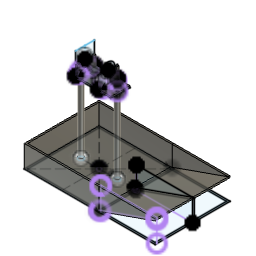
MiniFountain (Autodesk Fusion 360 design; units mm, degrees)
Autodesk Fusion 360 part; units mm, degrees
sketch "Base" plane through (0, 0, 0) normal (0, 0, 1) x (1, 0, 0)
  line L0 (70, 70) -> (-70, 70)
  line L1 (-70, 70) -> (-70, -70)
  line L2 (-70, -70) -> (70, -70)
  line L3 (70, -70) -> (70, 70)
  line L4 (70, 70) -> (-70, -70) construction
  line L5 (-70, 70) -> (70, -70) construction
  line L6 (-73.35, -73.35) -> (73.35, -73.35)
  line L7 (73.35, -73.35) -> (73.35, 73.35)
  line L8 (73.35, 73.35) -> (-73.35, 73.35)
  line L9 (-73.35, 73.35) -> (-73.35, -73.35)
  line L10 (70, 70) -> (180, 70)
  line L11 (70, -70) -> (180, -70)
  line L12 (180, -70) -> (180, 70)
  line L13 (70, 73.35) -> (183.35, 73.35)
  line L14 (183.35, -73.35) -> (183.35, 73.35)
  line L15 (70, -73.35) -> (183.35, -73.35)
  line L16 (0, 0) -> (-30.5813, 0)
  line L17 (0, 70) -> (0, -70) construction
  line L18 (0, 0) -> (30.5813, 0)
  circle A0 centre (-35.5812, 0.0143) radius 5
  circle A1 centre (35.5812, 0.0143) radius 5
  dimension "d5" = 140
  dimension "d6" = 140
  dimension "d8" = 3.35
  dimension "d9" = 110
  dimension "d10" = 110
  dimension "d16" = 30.5813
  dimension "d17" = 10
  constraint horizontal L0
  constraint perpendicular L0 L1
  constraint parallel L0 L2
  constraint parallel L1 L3
  constraint coincident L4 L16.start
  constraint coincident L5 L16.start
  constraint coincident L16.start L18.start
  constraint perpendicular L7 L10
  constraint perpendicular L7 L11
  constraint parallel L8 L16
  constraint midpoint L0 L17.start
  constraint midpoint L2 L17.end
  constraint symmetric L16.start L17 L18.start
  constraint symmetric L16.end L17 L18.end
  constraint coincident L16.end A0
  constraint symmetric L17 A0 A1
  measures "d5" distance of L1.end L2.end
  measures "d6" distance of L0.end L1.end
  measures "d9" distance of L0.start L10.end
  measures "d10" distance of L2.end L11.end
  measures "d16" distance of L16.start L16.end
  measures "d17" diameter of A0
extrude "Extrude1" add sketch "Base" along normal blind 43.35 contours L0 L1 L2 L6 L7 L8 L9 L10 L11 L13 L15 makes body 1
extrude "Extrude2" add sketch "Base" along normal blind 3.35 contours L0 L1 L2 L3 bodies 1
extrude "Extrude3" add sketch "Base" along normal blind 150 contours A0 | A1 bodies 1
sketch "Centered ramp wall" plane through (0, 0, 0) normal (0, 1, 0) x (1, 0, 0)
  line L0 (70, 0) -> (183.35, 0)
  line L1 (183.35, 0) -> (183.35, -43.35)
  line L2 (186.7, 0) -> (186.7, -43.35)
  line L3 (186.7, 0) -> (183.35, 0)
  line L4 (186.7, -43.35) -> (183.35, -43.35)
  line L5 (73.35, 0) -> (73.35, -43.35)
  line L6 (73.35, 0) -> (73.35, -43.35)
  line L7 (73.35, -43.35) -> (183.35, -43.35)
  line L8 (70, 0) -> (70, -3.35)
  line L9 (70, -3.35) -> (70, 0)
  line L10 (70, -3.35) -> (183.35, -43.35)
  line L11 (70, 0) -> (183.35, -40)
  dimension "d24" = 43.35
  constraint coincident L0.end L1.start
  constraint perpendicular L0 L1
  constraint perpendicular L1 L3
  constraint perpendicular L1 L4
  constraint coincident L5.start L6.start
  constraint coincident L5.end L6.end
  constraint coincident L8.end L9.start
  constraint coincident L0.start L8.start
  constraint coincident L1 L11.end
  constraint parallel L10 L11
  measures "d24" distance of L0.end L1.end
extrude "Extrude4" add sketch "Centered ramp wall" along normal mid plane 140 contours L5 L6 L8 L9 L10 L11 | L1 L5 L6 L10 L11 bodies 1
ref_plane "WorkPlane1" through (128.35, -70, 23.9411) normal (0, 1, 0) x (1, 0, 0)
sketch "ramp wall" plane through (129, -70, 24.7018) normal (0, 1, 0) x (1, 0, 0)
  line L0 (-55.65, -18.6482) -> (54.35, -18.6482)
  line L1 (54.35, 24.7018) -> (54.35, -18.6482)
  line L2 (-59, 24.7018) -> (54.35, -15.2982)
  line L3 (-55.65, 24.7018) -> (-55.65, -18.6482)
extrude "Extrude5" add sketch "ramp wall" against normal blind 3.35 separate body makes body 2
mirror "Mirror1" about plane through (0, 0, 0) normal (0, 1, 0) of bodies 2 makes body 3
sketch "top base" plane through (0, 0, 150) normal (0, 0, 1) x (-1, 0, 0)
  circle A0 centre (35.5812, -0.0143) radius 5
  circle A1 centre (-35.5812, -0.0143) radius 5
  circle A2 centre (35.5812, -0.0143) radius 5
  line L0 (42.0375, -18.425) -> (-42.0375, -18.425)
  line L1 (-42.0375, -18.425) -> (-42.0375, 18.425)
  line L2 (-42.0375, 18.425) -> (42.0375, 18.425)
  line L3 (42.0375, 18.425) -> (42.0375, -18.425)
  line L4 (42.0375, -18.425) -> (-42.0375, 18.425) construction
  line L5 (-42.0375, -18.425) -> (42.0375, 18.425) construction
  circle A3 centre (35.5812, -0.0143) radius 1.395
  circle A4 centre (-35.5812, -0.0143) radius 1.395
  dimension "d34" = 84.075
  dimension "d35" = 36.85
  dimension "d38" = 2.79
  dimension "d39" = 2.79
  constraint horizontal L0
  constraint perpendicular L0 L1
  constraint parallel L0 L2
  constraint parallel L1 L3
  constraint coincident L4 origin
  constraint coincident L5 origin
  constraint concentric A2 A3
  constraint concentric A1 A4
  measures "d34" distance of L1.end L2.end
  measures "d35" distance of L0.end L1.end
  measures "d38" diameter of A3
  measures "d39" diameter of A4
extrude "Extrude6" add sketch "top base" along normal blind 3.35 separate body contours A0 A2 | L0 L1 L2 L3 | A3 makes body 4
extrude "Extrude7" add 1 faces at (34.5421, -1.2887, 150) along direction (0, 0, 1) blind 3.35 on bodies 1 bodies 1 4
ref_plane "WorkPlane2" through (-27.7381, 0, 0) normal (1, 0, 0) x (0, 1, 0)
sketch "small holder" plane through (-27.7381, 0, 0) normal (1, 0, 0) x (0, 1, 0)
  line L0 (18.425, 153.35) -> (-18.425, 153.35)
  line L1 (0, 153.35) -> (11.955, 153.35)
  line L2 (11.955, 153.35) -> (18.955, 153.35)
  line L3 (0, 153.35) -> (0, 178.8174) construction
  circle A0 centre (0, 173.045) radius 12.165
  line L4 (0.0651, 185.2098) -> (0.0651, 195.7998)
  line L5 (18.425, 153.35) -> (18.425, 195.7998)
  line L6 (18.425, 195.7998) -> (0.0651, 195.7998)
  line L7 (-18.425, 153.35) -> (-18.425, 195.7998)
  line L8 (-18.425, 195.7998) -> (0.0651, 195.7998)
  line L9 (0, 173.045) -> (-18.425, 173.045)
  line L10 (0, 160.88) -> (0, 153.35)
  line L11 (0, 173.045) -> (18.425, 173.045)
  dimension "d48" = 24.33
  dimension "d52" = 7.53
  constraint midpoint L0 L1.start
  constraint parallel L0 L1
  constraint parallel L0 L2
  constraint perpendicular L1 L3
  constraint coincident A0 L4.start
  constraint vertical L4
  constraint coincident L0.start L5.start
  constraint perpendicular L0 L5
  constraint perpendicular L5 L6
  constraint coincident L0.end L7.start
  constraint perpendicular L0 L7
  constraint perpendicular L4 L8
  constraint coincident A0.centre L9.start
  constraint coincident L7 L9.end
  constraint perpendicular L7 L9
  constraint coincident A0 L10.start
  constraint coincident L3 L10.start
  constraint coincident L5 L11.end
  constraint perpendicular L5 L11
  measures "d48" diameter of A0
  measures "d52" distance of L1.start L10.start
ref_plane "WorkPlane3" through (17.2619, 0, 166.9625) normal (1, 0, 0) x (0, 1, 0)
sketch "big holder" plane through (17.2619, 0, 174.8999) normal (1, 0, 0) x (0, 1, 0)
  line L0 (18.425, -21.5499) -> (-18.425, -21.5499)
  line L1 (0, -21.5499) -> (0, -11.5499)
  circle A0 centre (0, 1.8501) radius 13.4
  line L2 (0, 1.8501) -> (-18.425, 1.8501)
  line L3 (-18.425, 1.8501) -> (-18.425, -21.5499)
  line L4 (18.425, -21.5499) -> (18.425, 1.8501)
  line L5 (18.425, 1.8501) -> (0, 1.8501)
  point P0 (18.425, -21.5499)
  point P1 (-18.425, -21.5499)
  dimension "d53" = 10
  dimension "d54" = 26.8
  constraint coincident P0 L0.start
  constraint coincident P1 L0.end
  constraint midpoint L0 L1.start
  constraint perpendicular L0 L1
  constraint coincident L1.end A0
  constraint coincident A0.centre L2.start
  constraint parallel L0 L2
  constraint perpendicular L0 L3
  constraint perpendicular L0 L4
  constraint perpendicular L4 L5
  measures "d53" distance of L1.start L1.end
  measures "d54" diameter of A0
extrude "Extrude8" add sketch "small holder" along normal blind 3.35 contours L0 L1 L2 A0 L5 L10 L11 | L0 A0 L7 L9 L10 bodies 1
extrude "Extrude9" add sketch "big holder" along normal blind 3.35 contours L0 L1 A0 L4 L5 | L0 L1 A0 L2 L3 bodies 1
sketch "top base hole" plane through (0, 0, 153.35) normal (0, 0, 1) x (-1, 0, 0)
  line L0 (-17.2619, 18.425) -> (-17.2619, -18.425)
  line L1 (-17.2619, -18.425) -> (24.3881, -18.425)
  line L2 (24.3881, -18.425) -> (24.3881, 18.425)
  line L3 (24.3881, 18.425) -> (-17.2619, 18.425)
  line L4 (-20.6119, -13.4) -> (-20.6119, 13.4)
  circle A0 centre (-7.6119, 0) radius 3.35
  line L5 (27.7381, 12.165) -> (27.7381, -12.165)
  line L6 (27.7381, 0) -> (-4.2619, 0) construction
  dimension "d61" = 6.7
  dimension "d64" = 32
  constraint midpoint L5 L6.start
  constraint coincident A0 L6.end
  constraint perpendicular L5 L6
  measures "d61" diameter of A0
  measures "d64" distance of L6.start L6.end
extrude "Extrude10" cut sketch "top base hole" against normal blind 3.35 contours A0 bodies 1
sketch "Projection_Back" plane through (0, 73.35, 0) normal (0, 1, 0) x (-1, 0, 0)
  line L0 (-73.35, 0) -> (73.35, 0)
  line L1 (73.35, 0) -> (73.35, 43.35)
  line L2 (73.35, 43.35) -> (-73.35, 43.35)
  line L3 (-73.35, 43.35) -> (-183.35, 43.35)
  line L4 (-183.35, 43.35) -> (-183.35, 40)
  line L5 (-183.35, 40) -> (-73.35, 1.1822)
  line L6 (-73.35, 1.1822) -> (-73.35, 0)
  line L7 (-183.35, 43.35) -> (-183.35, 40)
  line L8 (73.35, 43.35) -> (73.35, 0)
  constraint coincident L5.end L6.start
  constraint coincident L0.start L6.end
  constraint coincident L3.end L4.start
  constraint coincident L4.end L5.start
  constraint coincident L1.end L2.start
  constraint coincident L0.end L1.start
sketch "Projection_Front" plane through (0, -73.35, 0) normal (0, -1, 0) x (1, 0, 0)
  line L0 (-73.35, 0) -> (73.35, 0)
  line L1 (73.35, 43.35) -> (-73.35, 43.35)
  line L2 (-73.35, 43.35) -> (-73.35, 0)
  line L3 (183.35, 43.35) -> (73.35, 43.35)
  line L4 (73.35, 1.1822) -> (183.35, 40)
  line L5 (183.35, 40) -> (183.35, 43.35)
  line L6 (73.35, 1.1822) -> (73.35, 0)
  line L7 (183.35, 43.35) -> (183.35, 40)
  line L8 (-73.35, 43.35) -> (-73.35, 0)
  constraint coincident L4.start L6.start
  constraint coincident L0.end L6.end
  constraint coincident L3.start L5.end
  constraint coincident L4.end L5.start
  constraint coincident L1.end L2.start
  constraint coincident L0.start L2.end
sketch "Projection_Left" plane through (-73.35, 0, 0) normal (-1, 0, 0) x (0, -1, 0)
  line L0 (-73.35, 0) -> (73.35, 0)
  line L1 (73.35, 0) -> (73.35, 43.35)
  line L2 (73.35, 43.35) -> (-73.35, 43.35)
  line L3 (-73.35, 43.35) -> (-73.35, 0)
  line L4 (18.425, 173.045) -> (12.165, 173.045)
  arc A0 (-12.165, 173.045) -> (12.165, 173.045) centre (0, 173.045) ccw
  line L5 (-12.165, 173.045) -> (-18.425, 173.045)
  line L6 (-18.425, 173.045) -> (-18.425, 153.35)
  line L7 (-18.425, 153.35) -> (18.425, 153.35)
  line L8 (18.425, 153.35) -> (18.425, 173.045)
sketch "Projection_right" plane through (20.6119, 0, 0) normal (1, 0, 0) x (0, 1, 0)
  line L0 (18.425, 153.35) -> (18.425, 176.75)
  line L1 (18.425, 176.75) -> (13.4, 176.75)
  arc A0 (-13.4, 176.75) -> (13.4, 176.75) centre (0, 176.75) ccw
  line L2 (-13.4, 176.75) -> (-18.425, 176.75)
  line L3 (-18.425, 176.75) -> (-18.425, 153.35)
  line L4 (-18.425, 153.35) -> (18.425, 153.35)
sketch "Projection_Ramp" plane through (6.7006, 0, -18.9877) normal (-0.332777, 0, 0.943006) x (0, -1, 0)
  line L0 (70, 187.326) -> (-70, 187.326)
  line L1 (-70, 187.326) -> (-70, 70.6777)
  line L2 (-70, 70.6777) -> (-70, 67.1252)
  line L3 (-70, 67.1252) -> (70, 67.1252)
  line L4 (70, 67.1252) -> (70, 70.6777)
  line L5 (70, 70.6777) -> (70, 187.326)
sketch "Projection_Base" plane through (0, 0, 3.35) normal (0, 0, 1) x (-1, 0, 0)
  circle A0 centre (-35.5812, -0.0143) radius 5
  circle A1 centre (35.5812, -0.0143) radius 5
  line L0 (-70, 70) -> (-70, -70)
  line L1 (-70, -70) -> (70, -70)
  line L2 (70, -70) -> (70, 70)
  line L3 (70, 70) -> (-70, 70)
sketch "Projection_Top" plane through (0, 0, 153.35) normal (0, 0, 1) x (-1, 0, 0)
  circle A0 centre (-7.6119, 0) radius 3.35
  line L0 (-17.2619, -18.425) -> (24.3881, -18.425)
  line L1 (24.3881, 18.425) -> (-17.2619, 18.425)
  circle A1 centre (-7.6119, 0) radius 3.35
  line L2 (-42.0375, 18.425) -> (42.0375, 18.425)
  line L3 (42.0375, 18.425) -> (42.0375, -18.425)
  line L4 (42.0375, -18.425) -> (-42.0375, -18.425)
  line L5 (-42.0375, -18.425) -> (-42.0375, 18.425)
  circle A2 centre (-35.5812, -0.0143) radius 5
  circle A3 centre (35.5812, -0.0143) radius 5
  circle A4 centre (35.5812, -0.0143) radius 5
  line L6 (27.7381, -18.425) -> (42.0375, -18.425)
  line L7 (42.0375, -18.425) -> (42.0375, 18.425)
  line L8 (42.0375, 18.425) -> (27.7381, 18.425)
  circle A5 centre (-35.5812, -0.0143) radius 5
sketch "Projection_Left_Acrylic" plane through (-73.35, 0, 0) normal (-1, 0, 0) x (0, -1, 0)
  line L0 (-73.35, 0) -> (73.35, 0)
  line L1 (73.35, 0) -> (73.35, 43.35)
  line L2 (73.35, 43.35) -> (-73.35, 43.35)
  line L3 (-73.35, 43.35) -> (-73.35, 0)
sketch "Projection_small" plane through (-27.7381, 0, 0) normal (-1, 0, 0) x (0, -1, 0)
  line L0 (18.425, 173.045) -> (12.165, 173.045)
  arc A0 (-12.165, 173.045) -> (12.165, 173.045) centre (0, 173.045) ccw
  line L1 (-12.165, 173.045) -> (-18.425, 173.045)
  line L2 (-18.425, 173.045) -> (-18.425, 153.35)
  line L3 (-18.425, 153.35) -> (18.425, 153.35)
  line L4 (18.425, 153.35) -> (18.425, 173.045)
equation "base_size = 140 mm"
equation "base_walls = 40 mm"
equation "collector_length = 110 mm"
equation "height = 150 mm"
equation "d5 = base_size"
equation "d6 = base_size"
equation "thickness = 3.35 mm"
equation "d8 = thickness"
equation "d9 = collector_length"
equation "d11 = -thickness"
equation "pump_length = 58.25 mm"
equation "pump_short_diameter = 24.33 mm"
equation "pump_long_diameter = 26.80 mm"
equation "rod_diameter = 10 mm"
equation "d16 = ( pump_length / 2 ) * 1.05"
equation "d17 = rod_diameter"
equation "d18 = base_walls + thickness"
equation "d20 = thickness"
equation "d22 = height"
equation "d24 = thickness + base_walls"
equation "d25 = -thickness"
equation "d27 = base_size / 2"
equation "d29 = -base_size / 2"
equation "d30 = -thickness"
equation "d34 = pump_length * 1.1 + rod_diameter * 2"
equation "d35 = pump_long_diameter + thickness * 3"
equation "screw_diameter = 3 mm"
equation "laser_kerf = 0.21 mm"
equation "d38 = screw_diameter - laser_kerf"
equation "d39 = screw_diameter - laser_kerf"
equation "d40 = thickness"
equation "d42 = thickness"
equation "d44 = -pump_length / 2.1"
equation "d48 = pump_short_diameter"
equation "d52 = 10 mm - ( pump_long_diameter - pump_short_diameter )"
equation "d54 = pump_long_diameter"
equation "d55 = thickness"
equation "d57 = thickness"
equation "rubber_tube_diameter = 6.70 mm"
equation "d61 = rubber_tube_diameter"
equation "d62 = -thickness"
